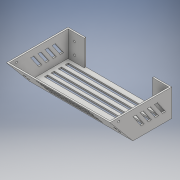
# Autodesk Inventor part: Chassi_Front
Saved by Autodesk Inventor 2018.2 (Build 222227000, 227)
## iProperties
Created: 2018-08-12
Part Number: Chassi_Front
Material: Generic
Document SubType Name: Modeling
Designer: mateu
Density: 1 g/cm^3
Appearance: Default
Author: mateu
Autodesk Inventor part; units mm, degrees
ref_plane "YZ Plane" through (0, 0, 0) normal (1, 0, 0) x (0, 1, 0)
ref_plane "XY Plane" through (0, 0, 0) normal (0, 0, 1) x (1, 0, 0)
sketch "Sketch1" plane through (0, 0, 0) normal (0, 0, 1) x (1, 0, 0)
  line L0 (0, 0) -> (160, 0)
  line L1 (160, 0) -> (160, 60)
  line L2 (160, 60) -> (0, 60)
  line L3 (0, 60) -> (0, 0)
  line L4 (8.5291, 51.8697) -> (148.5291, 51.8697)
  line L5 (148.5291, 51.8697) -> (148.5291, 46.8697)
  line L6 (148.5291, 46.8697) -> (8.5291, 46.8697)
  line L7 (8.5291, 46.8697) -> (8.5291, 51.8697)
  line L8 (8.5291, 41.2311) -> (148.5291, 41.2311)
  line L9 (148.5291, 41.2311) -> (148.5291, 36.2311)
  line L10 (148.5291, 36.2311) -> (8.5291, 36.2311)
  line L11 (8.5291, 36.2311) -> (8.5291, 41.2311)
  line L12 (8.5291, 30) -> (148.5291, 30)
  line L13 (148.5291, 30) -> (148.5291, 25)
  line L14 (148.5291, 25) -> (8.5291, 25)
  line L15 (8.5291, 25) -> (8.5291, 30)
  line L16 (8.5291, 19.9539) -> (148.5291, 19.9539)
  line L17 (148.5291, 19.9539) -> (148.5291, 14.9539)
  line L18 (148.5291, 14.9539) -> (8.5291, 14.9539)
  line L19 (8.5291, 14.9539) -> (8.5291, 19.9539)
  dimension "d0" = 160
  dimension "d1" = 60
  dimension "d2" = 140
  dimension "d3" = 5
  dimension "d4" = 5
  dimension "d5" = 5
  dimension "d6" = 5
  constraints: 40 end point, 10 parallel, 6 point on line, 5 horizontal, 5 perpendicular
  measures "d0" distance of L2.end L1.end
  measures "d1" distance of L1.end L0.end
  measures "d2" distance of L5.end L6.end
  measures "d3" distance of L4.end L5.end
  measures "d4" distance of L8.end L9.end
  measures "d5" distance of L12.end L13.end
  measures "d6" distance of L16.end L17.end
extrude "Extrusion1" add sketch "Sketch1" along normal blind 2.4
sketch "Sketch2" plane through (0, 0, 2.4) normal (0, 0, 1) x (1, 0, 0)
  line L0 (0, 60) -> (0, 0) projected
  line L1 (0, 0) -> (160, 0) projected
  line L2 (0, 60) -> (2.4, 60)
  line L3 (2.4, 60) -> (2.4, 0)
  line L4 (2.4, 0) -> (0, 0)
  line L5 (0, 0) -> (0, 60)
  line L6 (160, 60) -> (0, 60) projected
  line L7 (160, 0) -> (157.6, 0)
  line L8 (157.6, 0) -> (157.6, 60)
  line L9 (157.6, 60) -> (160, 60)
  line L10 (160, 60) -> (160, 0)
  dimension "d9" = 2.4
  dimension "d10" = 2.4
  constraints: 16 end point, 4 parallel, 2 horizontal, 2 perpendicular, 2 point on line
  measures "d9" distance of L3.end L4.end
  measures "d10" distance of L8.end L9.end
extrude "Extrusion2" add sketch "Sketch2" along normal blind 39.6 contours L2 L3 L1 L0 | L6 L10 L1 L8
sketch "Sketch3" plane through (160, 0, 0) normal (1, 0, 0) x (0, 0, -1)
  line L0 (0, 0) -> (-42, -35.2422)
  line L1 (0, 0) -> (54.8271, 0) construction
  line L2 (-42, 0) -> (-42, 60) projected
  line L3 (-42, -35.2422) -> (-42, 0)
  line L4 (-42, 0) -> (0, 0)
  dimension "d13" = 140
  constraints: 8 end point, 1 collinear, 1 equal length, 1 horizontal, 1 perpendicular
  measures "d13" angle of L0 L1
extrude "Extrusion3" add sketch "Sketch3" against normal blind 2.4
sketch "Sketch4" plane through (0, 0, 0) normal (-1, 0, 0) x (0, 0, 1)
  line L0 (0, 0) -> (42, 0) projected
  line L1 (42, 0) -> (0, 0)
  line L2 (0, 0) -> (42, -35.2422) projected
  line L3 (0, 0) -> (42, -35.2422)
  line L4 (42, -35.2422) -> (42, 0)
  constraints: 6 end point, 2 collinear, 1 perpendicular
extrude "Extrusion4" add sketch "Sketch4" against normal blind 2.4
sketch "Sketch5" plane through (157.6, 0, 2.4) normal (-1, 0, 0) x (0, 0, 1)
  line L0 (-2.4, 0) -> (0, 0)
  line L1 (39.6, 60) -> (39.6, -35.2422) projected
  line L2 (39.6, -35.2422) -> (39.6, -32.8422)
  line L3 (39.6, -32.8422) -> (0, 0)
  line L4 (-2.4, 0) -> (39.6, -35.2422)
  dimension "d18" = 2.4
  constraints: 8 end point, 1 horizontal, 1 point on line
  measures "d18" distance of L1.end L2.end
extrude "Extrusion5" add sketch "Sketch5" along normal blind 157.6
sketch "Sketch6" plane through (160, 60, 42) normal (1, 0, 0) x (0, 0, -1)
  line L0 (10, -60) -> (10, -55)
  line L1 (10, -49) -> (10, -44)
  line L2 (10, -38) -> (10, -33)
  line L3 (10, -27) -> (10, -22)
  line L4 (10, -22) -> (28.0953, -9.4875)
  line L5 (28.0953, -9.4875) -> (28.0953, -14.4875)
  line L6 (42, 0) -> (0, 0) projected
  line L7 (28.0953, -20.4875) -> (28.0953, -25.4875)
  line L8 (28.0953, -31.4875) -> (28.0953, -36.4875)
  line L9 (28.0953, -42.4875) -> (28.0953, -47.4875)
  line L10 (28.0953, -47.4875) -> (10, -60)
  line L11 (28.0953, -42.4875) -> (10, -55)
  line L12 (28.0953, -36.4875) -> (10, -49)
  line L13 (10, -44) -> (28.0953, -31.4875)
  line L14 (28.0953, -25.4875) -> (10, -38)
  line L15 (10, -33) -> (28.0953, -20.4875)
  line L16 (28.0953, -14.4875) -> (10, -27)
  line L17 (0, -95.2422) -> (0, 0) projected
  circle A0 centre (5, -81.9088) radius 1.5
  line L18 (42, -60) -> (0, -95.2422) projected
  dimension "d21" = 5
  dimension "d22" = 6
  dimension "d23" = 5
  dimension "d24" = 6
  dimension "d25" = 5
  dimension "d26" = 6
  dimension "d27" = 5
  dimension "d28" = 22
  dimension "d29" = 5
  dimension "d30" = 6
  dimension "d31" = 5
  dimension "d32" = 6
  dimension "d33" = 5
  dimension "d34" = 6
  dimension "d35" = 5
  dimension "d36" = 10
  dimension "d77" = 3
  dimension "d78" = 7
  dimension "d79" = 5
  constraints: 32 end point, 6 point on line, 1 centre point, 1 parallel, 1 perpendicular, 1 vertical
  measures "d21" distance of L0.start L0.end
  measures "d22" distance of L0.end L1.start
  measures "d23" distance of L1.start L1.end
  measures "d24" distance of L1.end L2.start
  measures "d25" distance of L2.start L2.end
  measures "d26" distance of L2.end L3.start
  measures "d27" distance of L3.start L3.end
  measures "d28" distance of L3.end L4.end
  measures "d29" distance of L4.end L5.end
  measures "d30" distance of L5.end L7.start
  measures "d31" distance of L7.start L7.end
  measures "d32" distance of L7.end L8.start
  measures "d33" distance of L8.start L8.end
  measures "d34" distance of L8.end L9.start
  measures "d35" distance of L9.start L9.end
  measures "d36" distance between parallel lines of L17 L1
  measures "d77" diameter of A0
  measures "d78" distance from line of L18 A0.centre
  measures "d79" distance from line of L17 A0.centre
ref_plane "Work Plane1" through (0, -50, 0) normal (0, 1, 0) x (-1, 0, 0)
sketch "Sketch7" plane through (0, -50, 0) normal (0, 1, 0) x (-1, 0, 0)
  circle A0 centre (-10, 20) radius 2
  line L0 (-157.6, 42) -> (-2.4, 42) projected
  line L1 (-80, 42) -> (-80, 0)
  line L2 (-8.5291, 0) -> (-148.5291, 0) projected
  circle A1 centre (-150, 20) radius 2
  line L3 (-160, 0) -> (-160, 42) projected
  line L4 (0, 0) -> (0, 42) projected
  line L5 (0, 0) -> (-160, 0) projected
  line L6 (-80, 35.2897) -> (-40, 35.2897)
  line L7 (-40, 35.2897) -> (-40, 31.2897)
  line L8 (-40, 31.2897) -> (-120, 31.2897)
  line L9 (-120, 31.2897) -> (-120, 35.2897)
  line L10 (-120, 35.2897) -> (-80, 35.2897)
  line L11 (-39.9996, 27.2897) -> (-39.9998, 23.2897)
  line L12 (-40, 19.2897) -> (-40, 15.2897)
  line L13 (-40, 15.2897) -> (-120, 15.2897)
  line L14 (-120, 15.2897) -> (-120, 19.2897)
  line L15 (-120, 19.2897) -> (-40, 19.2897)
  line L16 (-39.9998, 23.2897) -> (-120, 23.2897)
  line L17 (-120, 23.2897) -> (-120, 27.2897)
  line L18 (-120, 27.2897) -> (-39.9996, 27.2897)
  line L19 (-40.1762, 11.5108) -> (-40.1762, 7.5108)
  line L20 (-40.1762, 7.5108) -> (-120.1762, 7.5108)
  line L21 (-120.1762, 7.5108) -> (-120.1762, 11.5108)
  line L22 (-120.1762, 11.5108) -> (-40.1762, 11.5108)
  dimension "d40" = 4
  dimension "d41" = 4
  dimension "d42" = 10
  dimension "d43" = 10
  dimension "d44" = 20
  dimension "d45" = 20
  dimension "d46" = 40
  dimension "d47" = 4
  dimension "d49" = 4
  dimension "d50" = 4
  dimension "d51" = 4
  dimension "d52" = 4
  dimension "d55" = 4
  dimension "d56" = 80
  dimension "d57" = 80
  dimension "d58" = 80
  dimension "d59" = 80.0002
  dimension "d60" = 80
  constraints: 36 end point, 8 point on line, 7 perpendicular, 4 horizontal, 2 centre point, 2 vertical, 1 midpoint, 1 parallel
  measures "d40" diameter of A0
  measures "d41" diameter of A1
  measures "d42" distance from line of L3 A1.centre
  measures "d43" distance from line of L4 A0.centre
  measures "d44" distance from line of L5 A0.centre
  measures "d45" distance from line of L5 A1.centre
  measures "d46" distance of L6.start L6.end
  measures "d47" distance of L6.end L7.end
  measures "d49" distance of L7.end L11.start
  measures "d50" distance of L11.start L11.end
  measures "d51" distance of L11.end L12.start
  measures "d52" distance of L12.start L12.end
  measures "d55" distance of L19.start L19.end
  measures "d56" distance of L19.end L20.end
  measures "d57" distance of L12.end L13.end
  measures "d58" distance of L14.end L12.start
  measures "d59" distance of L11.end L16.end
  measures "d60" distance of L7.end L8.end
extrude "Extrusion8" cut sketch "Sketch7" along normal blind 160
sketch "Sketch8" plane through (0, -35.2422, 42) normal (0, -0.7660444, -0.6427876) x (1, 0, 0)
  circle A0 centre (10, -37.8271) radius 2
  line L0 (0, -54.8271) -> (0, 0) projected
  circle A1 centre (150, -37.8271) radius 2
  line L1 (160, -54.8271) -> (160, 0) projected
  line L2 (0, -54.8271) -> (160, -54.8271) projected
  dimension "d63" = 4
  dimension "d64" = 10
  dimension "d65" = 4
  dimension "d66" = 10
  dimension "d67" = 17
  dimension "d68" = 17
  constraints: 2 centre point
  measures "d63" diameter of A0
  measures "d64" distance from line of L0 A0.centre
  measures "d65" diameter of A1
  measures "d66" distance from line of L1 A1.centre
  measures "d67" distance from line of L2 A0.centre
  measures "d68" distance from line of L2 A1.centre
extrude "Extrusion9" cut sketch "Sketch8" against normal blind 160
sketch "Sketch9" plane through (157.6, 60, 2.4) normal (-1, 0, 0) x (0, 0, 1)
  line L0 (39.6, 0) -> (39.6, -92.8422) projected
  line L1 (0, 0) -> (39.6, 0)
  line L2 (39.6, 0) -> (39.6, -2.4)
  line L3 (39.6, -2.4) -> (0, -2.4)
  line L4 (0, -2.4) -> (0, 0)
  point P0 (-2.4, -60)
  dimension "d71" = 2.4
  constraints: 8 end point, 2 parallel, 1 horizontal, 1 perpendicular, 1 point on line
  measures "d71" distance of L1.end L2.end
extrude "Extrusion10" add sketch "Sketch9" along normal blind 25
sketch "Sketch10" plane through (2.4, 60, 42) normal (1, 0, 0) x (0, 0, -1)
  line L0 (39.6, 0) -> (0, 0) projected
  line L1 (0, 0) -> (0, -92.8422) projected
  line L2 (39.6, 0) -> (0, 0)
  line L3 (0, 0) -> (0, -2.4)
  line L4 (0, -2.4) -> (39.6, -2.4)
  line L5 (39.6, -2.4) -> (39.6, 0)
  point P0 (42, -60)
  dimension "d74" = 2.4
  constraints: 8 end point, 2 parallel, 1 horizontal, 1 perpendicular, 1 point on line
  measures "d74" distance of L3.end L2.end
extrude "Extrusion11" add sketch "Sketch10" along normal blind 25
extrude "Extrusion12" cut sketch "Sketch6" against normal blind 160
sketch "Sketch11" plane through (0, 60, 0) normal (0, 1, 0) x (1, 0, 0)
  circle A0 centre (147.5, -30) radius 1.5
  line L0 (160, 0) -> (160, -42) projected
  line L1 (160, -42) -> (132.6, -42) projected
  circle A1 centre (147.5, -12) radius 1.5
  line L2 (160, 0) -> (0, 0) projected
  circle A2 centre (12.5, -30) radius 1.5
  circle A3 centre (12.5, -12) radius 1.5
  line L3 (0, 0) -> (0, -42) projected
  line L4 (0, -42) -> (27.4, -42) projected
  line L5 (141.6, -29.5) -> (139.6, -29.5)
  line L6 (139.6, -29.5) -> (139.6, -12.5)
  line L7 (139.6, -12.5) -> (141.6, -12.5)
  line L8 (141.6, -12.5) -> (141.6, -29.5)
  line L9 (132.6, -42) -> (132.6, -2.4) projected
  line L10 (20.4, -29.5) -> (18.4, -29.5)
  line L11 (18.4, -29.5) -> (18.4, -12.5)
  line L12 (18.4, -12.5) -> (20.4, -12.5)
  line L13 (20.4, -12.5) -> (20.4, -29.5)
  line L14 (27.4, -2.4) -> (27.4, -42) projected
  dimension "d82" = 3
  dimension "d83" = 12.5
  dimension "d84" = 12
  dimension "d85" = 3
  dimension "d86" = 12.5
  dimension "d87" = 12
  dimension "d88" = 3
  dimension "d89" = 3
  dimension "d90" = 12.5
  dimension "d91" = 12
  dimension "d92" = 12
  dimension "d93" = 12.5
  dimension "d96" = 7
  dimension "d97" = 2
  dimension "d98" = 12.5
  dimension "d99" = 12.5
  dimension "d101" = 2
  dimension "d103" = 7
  dimension "d104" = 12.5
  dimension "d107" = 12.5
  constraints: 16 end point, 4 centre point, 4 parallel, 2 horizontal, 2 perpendicular
  measures "d82" diameter of A0
  measures "d83" distance from line of L0 A0.centre
  measures "d84" distance from line of L1 A0.centre
  measures "d85" diameter of A1
  measures "d86" distance from line of L0 A1.centre
  measures "d87" distance from line of L2 A1.centre
  measures "d88" diameter of A2
  measures "d89" diameter of A3
  measures "d90" distance from line of L3 A3.centre
  measures "d91" distance from line of L2 A3.centre
  measures "d92" distance from line of L4 A2.centre
  measures "d93" distance from line of L3 A2.centre
  measures "d96" distance between parallel lines of L9 L6
  measures "d97" distance of L5.start L5.end
  measures "d98" distance between parallel lines of L2 L7
  measures "d99" distance between parallel lines of L1 L5
  measures "d101" distance of L11.end L12.end
  measures "d103" distance between parallel lines of L14 L13
  measures "d104" distance between parallel lines of L4 L10
  measures "d107" distance from line of L2 L11.end
extrude "Extrusion13" cut sketch "Sketch11" against normal blind 12 contours A0 | A1 | A2 | A3
extrude "Extrusion14" add sketch "Sketch11" along normal blind 3 contours L5 L6 L7 L8 | L10 L11 L12 L13
equation "\"d42\" = d43"
equation "\"d45\" = d44"
equation "\"d66\" = d64"
equation "\"d68\" = d67"
equation "\"d86\" = d83"
equation "\"d87\" = d84"
equation "\"d90\" = d86"
equation "\"d91\" = d87"
equation "\"d92\" = d84"
equation "\"d93\" = d83"
equation "\"d103\" = d96"
equation "\"d104\" = d99"
equation "\"d107\" = d98"
body "Solid1"
